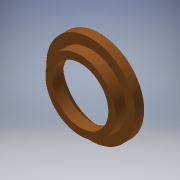
# Autodesk Inventor part: Seat
Saved by Autodesk Inventor 2018 (Build 220112000, 112)
## iProperties
Shininess: 64.0
Length Units: 11269
Angle Units: 11279
Time Units: 11290
Mass Units: 11283
Length Display Precision: 3
Angle Display Precision: 2
Compacted: True
Part Number: Seat
Document SubType Name: Modeling
Created: 2003-04-19
Designer: James M. Leake
Material: Bronze, Soft Tin
Density: 8.874 g/cm^3
Appearance: Bronze - Satin
Density: 0.0
Volumn: 0.0
Area: 0.0
PropertySet Name: Model Information
Control State: 0
Master: False
Checked Out: False
Author: James M. Leake
Autodesk Inventor part; units mm, degrees
ref_plane "YZ Plane" through (0, 0, 0) normal (1, 0, 0) x (0, 1, 0)
ref_plane "XZ Plane" through (0, 0, 0) normal (0, 1, 0) x (-1, 0, 0)
ref_plane "XY Plane" through (0, 0, 0) normal (0, 0, 1) x (1, 0, 0)
sketch "Sketch1" plane through (0, 0, 0) normal (0, 0, 1) x (1, 0, 0)
  line L0 (0, -8.5138) -> (0, 6.8862) projected
  line L1 (16, 3.5862) -> (16, -7.4138)
  line L2 (16, -7.4138) -> (20, -7.4138)
  line L3 (20, -7.4138) -> (20, -1.4138)
  line L4 (20, -1.4138) -> (25.5, -1.4138)
  line L5 (25.5, -1.4138) -> (25.5, 3.5862)
  line L6 (25.5, 3.5862) -> (16, 3.5862)
  dimension "d0" = 32
  dimension "d1" = 51
  dimension "d2" = 40
  dimension "d3" = 5
  dimension "d4" = 11
  constraints: 12 end point, 5 parallel, 1 horizontal, 1 perpendicular
  measures "d0" diameter of L1 L0
  measures "d1" diameter of L5 L0
  measures "d2" diameter of L3 L0
  measures "d3" distance of L4.end L5.end
  measures "d4" distance between parallel lines of L2 L6
revolve "Revolution1" add sketch "Sketch1" angle 360 about axis through (0, -10, 0) along (0, 1, 0)
chamfer "Chamfer1" distance 5 angle 45 1 edges at (-16, 3.5862, 0)
body "Solid1"
